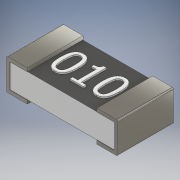
# Autodesk Inventor part: 21-1001
Saved by Autodesk Inventor 2018 (Build 220112000, 112)
## iProperties
Created: 2019-09-21
Part Number: 21-1001
Material: Copper
Document SubType Name: Modeling
Designer: Bradley
Density: 8.94 g/cm^3
Appearance: Smooth - White
Author: Bradley
Autodesk Inventor part; units mm, degrees
ref_plane "YZ Plane" through (0, 0, 0) normal (1, 0, 0) x (0, 1, 0)
ref_plane "XZ Plane" through (0, 0, 0) normal (0, 1, 0) x (-1, 0, 0)
ref_plane "XY Plane" through (0, 0, 0) normal (0, 0, 1) x (1, 0, 0)
sketch "Sketch1" plane through (0, 0, 0) normal (0, 1, 0) x (-1, 0, 0)
  line L0 (0.75, 0.175) -> (-0.75, 0.175)
  line L1 (-0.75, 0.175) -> (-0.75, -0.175)
  line L2 (-0.75, -0.175) -> (0.75, -0.175)
  line L3 (0.75, -0.175) -> (0.75, 0.175)
  line L4 (0.5, 0.175) -> (0.5, 0.225)
  line L5 (0.5, 0.225) -> (0.8, 0.225)
  line L6 (0.8, 0.225) -> (0.8, -0.225)
  line L7 (0.8, -0.225) -> (0.5, -0.225)
  line L8 (0.5, -0.225) -> (0.5, -0.175)
  line L9 (-0.5, 0.175) -> (-0.5, 0.225)
  line L10 (-0.5, 0.225) -> (-0.8, 0.225)
  line L11 (-0.8, 0.225) -> (-0.8, -0.225)
  line L12 (-0.8, -0.225) -> (-0.5, -0.225)
  line L13 (-0.5, -0.175) -> (-0.5, -0.225)
  line L14 (0.5, 0.175) -> (-0.5, 0.175)
  point P0 (0, 0)
  point P1 (0, 0.175)
  point P2 (0.75, 0)
  dimension "d0" = 1.6
  dimension "d1" = 0.05
  dimension "d2" = 0.05
  dimension "d3" = 0.45
  dimension "d4" = 0.3
  constraints: 30 end point, 12 point on line, 7 perpendicular, 3 collinear, 3 midpoint, 2 parallel, 1 horizontal, 1 horizontal alignment, 1 vertical, 1 vertical alignment
  measures "d0" distance between parallel lines of L11 L6
  measures "d1" distance of L7.end L8.end
  measures "d2" distance between parallel lines of L6 L3
  measures "d3" distance of L5.end L6.end
  measures "d4" distance of L6.end L7.end
extrude "Extrusion1" add sketch "Sketch1" along normal mid plane 0.8 contours L0 L4 L5 L6 L7 L8 L2 L3 | L0 L1 L2 L13 L12 L11 L10 L9
extrude "Extrusion2" add sketch "Sketch1" along normal mid plane 0.79 contours L3 L2 L1 L0
sketch "Sketch2" plane through (-0.5, -0.395, 0.175) normal (0, 0, 1) x (1, 0, 0)
  line L0 (0, 0) -> (0, 0.79) projected
  line L1 (1, 0) -> (0, 0) projected
  line L2 (1, 0) -> (1, 0.79) projected
  line L3 (0, 0.79) -> (1, 0.79) projected
  line L4 (0, 0.395) -> (1, 0.395) construction
  spline S0 degree 2 poles (0.3279, 0.395) (0.3279, 0.2874) (0.2653, 0.1866) (0.2002, 0.1866) knots 0 0 0 1 2 2 2
  spline S1 degree 2 poles (0.2002, 0.1866) (0.134, 0.1866) (0.0721, 0.2893) (0.0721, 0.3947) knots 0 0 0 1 2 2 2
  spline S2 degree 2 poles (0.0721, 0.3947) (0.0721, 0.5029) (0.1347, 0.6031) (0.2002, 0.6031) knots 0 0 0 1 2 2 2
  spline S3 degree 2 poles (0.2002, 0.6031) (0.266, 0.6031) (0.3279, 0.4994) (0.3279, 0.395) knots 0 0 0 1 2 2 2
  spline S4 degree 2 poles (0.2592, 0.2731) (0.2669, 0.2929) (0.2734, 0.3538) (0.2734, 0.395) knots 0 0 0 1 2 2 2
  spline S5 degree 2 poles (0.2734, 0.395) (0.2734, 0.4362) (0.2669, 0.4968) (0.2588, 0.5172) knots 0 0 0 1 2 2 2
  spline S6 degree 2 poles (0.2588, 0.5172) (0.2507, 0.5376) (0.2225, 0.5587) (0.2002, 0.5587) knots 0 0 0 1 2 2 2
  spline S7 degree 2 poles (0.2002, 0.5587) (0.1778, 0.5587) (0.1489, 0.5376) (0.1405, 0.5166) knots 0 0 0 1 2 2 2
  spline S8 degree 2 poles (0.1405, 0.5166) (0.1324, 0.4961) (0.1266, 0.4339) (0.1266, 0.3947) knots 0 0 0 1 2 2 2
  spline S9 degree 2 poles (0.1266, 0.3947) (0.1266, 0.3525) (0.1318, 0.2961) (0.1402, 0.2741) knots 0 0 0 1 2 2 2
  spline S10 degree 2 poles (0.1402, 0.2741) (0.148, 0.2533) (0.1768, 0.231) (0.2002, 0.231) knots 0 0 0 1 2 2 2
  spline S11 degree 2 poles (0.2002, 0.231) (0.2222, 0.231) (0.2511, 0.2521) (0.2592, 0.2731) knots 0 0 0 1 2 2 2
  line L5 (0.6057, 0.195) -> (0.4105, 0.195)
  line L6 (0.4105, 0.195) -> (0.4105, 0.2358)
  line L7 (0.4105, 0.2358) -> (0.4831, 0.2358)
  line L8 (0.4831, 0.2358) -> (0.4831, 0.5039)
  line L9 (0.4831, 0.5039) -> (0.4105, 0.5039)
  line L10 (0.4105, 0.5039) -> (0.4105, 0.5405)
  spline S12 degree 2 poles (0.4105, 0.5405) (0.4517, 0.5405) (0.4906, 0.5639) (0.4932, 0.5963) knots 0 0 0 1 2 2 2
  line L11 (0.4932, 0.5963) -> (0.5347, 0.5963)
  line L12 (0.5347, 0.5963) -> (0.5347, 0.2358)
  line L13 (0.5347, 0.2358) -> (0.6057, 0.2358)
  line L14 (0.6057, 0.2358) -> (0.6057, 0.195)
  spline S13 degree 2 poles (0.9282, 0.395) (0.9282, 0.2874) (0.8656, 0.1866) (0.8005, 0.1866) knots 0 0 0 1 2 2 2
  spline S14 degree 2 poles (0.8005, 0.1866) (0.7344, 0.1866) (0.6724, 0.2893) (0.6724, 0.3947) knots 0 0 0 1 2 2 2
  spline S15 degree 2 poles (0.6724, 0.3947) (0.6724, 0.5029) (0.735, 0.6031) (0.8005, 0.6031) knots 0 0 0 1 2 2 2
  spline S16 degree 2 poles (0.8005, 0.6031) (0.8663, 0.6031) (0.9282, 0.4994) (0.9282, 0.395) knots 0 0 0 1 2 2 2
  spline S17 degree 2 poles (0.8595, 0.2731) (0.8673, 0.2929) (0.8737, 0.3538) (0.8737, 0.395) knots 0 0 0 1 2 2 2
  spline S18 degree 2 poles (0.8737, 0.395) (0.8737, 0.4362) (0.8673, 0.4968) (0.8592, 0.5172) knots 0 0 0 1 2 2 2
  spline S19 degree 2 poles (0.8592, 0.5172) (0.8511, 0.5376) (0.8229, 0.5587) (0.8005, 0.5587) knots 0 0 0 1 2 2 2
  spline S20 degree 2 poles (0.8005, 0.5587) (0.7781, 0.5587) (0.7493, 0.5376) (0.7408, 0.5166) knots 0 0 0 1 2 2 2
  spline S21 degree 2 poles (0.7408, 0.5166) (0.7327, 0.4961) (0.7269, 0.4339) (0.7269, 0.3947) knots 0 0 0 1 2 2 2
  spline S22 degree 2 poles (0.7269, 0.3947) (0.7269, 0.3525) (0.7321, 0.2961) (0.7405, 0.2741) knots 0 0 0 1 2 2 2
  spline S23 degree 2 poles (0.7405, 0.2741) (0.7483, 0.2533) (0.7771, 0.231) (0.8005, 0.231) knots 0 0 0 1 2 2 2
  spline S24 degree 2 poles (0.8005, 0.231) (0.8225, 0.231) (0.8514, 0.2521) (0.8595, 0.2731) knots 0 0 0 1 2 2 2
  point P0 (0.5, 0.395)
  constraints: 2 end point, 2 midpoint, 1 horizontal
extrude "Extrusion3" add sketch "Sketch2" along normal blind 0.02 contours S0 S1 S2 S3 | L5 L6 L7 L8 L9 L10 S12 L11 L12 L13 L14 | S13 S14 S15 S16
fillet "Fillet1" radius 0.02 4 edges at (-0.8, 0, 0.225) (-0.8, 0, -0.225) (0.8, 0, 0.225) (0.8, 0, -0.225)
equation "\"d2\" = d1"
body "Solid1"
